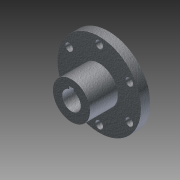
# Autodesk Inventor part: wheel hub
Saved by Autodesk Inventor 2011 SP1 (Build 150282100, 282)
## iProperties
Created: 2012-01-20
Part Number: wheel hub
Document SubType Name: Modeling
Designer: Christopher
Density: 1 g/cm^3
Author: Christopher
Autodesk Inventor part; units mm, degrees
ref_plane "YZ Plane" through (0, 0, 0) normal (1, 0, 0) x (0, 1, 0)
ref_plane "XZ Plane" through (0, 0, 0) normal (0, 1, 0) x (-1, 0, 0)
ref_plane "XY Plane" through (0, 0, 0) normal (0, 0, 1) x (1, 0, 0)
sketch "Sketch1" plane through (0, 0, 0) normal (0, 0, 1) x (1, 0, 0)
  circle A0 centre (0, 0) radius 28.575
  circle A1 centre (0, 0) radius 6.35
  line L0 (-1.5875, 4.7625) -> (1.5875, 4.7625)
  line L1 (1.5875, 4.7625) -> (1.5875, 7.9375)
  line L2 (1.5875, 7.9375) -> (-1.5875, 7.9375)
  line L3 (-1.5875, 7.9375) -> (-1.5875, 4.7625)
  line L4 (1.5875, 6.35) -> (-1.5875, 6.35)
  circle A2 centre (0, 0) radius 12.7
  point P0 (0, 4.7625)
  point P1 (0, 23.8125)
  point P2 (-20.6222, 11.9063)
  point P3 (-20.6222, -11.9062)
  point P4 (0, -23.8125)
  point P5 (20.6222, -11.9063)
  point P6 (20.6222, 11.9062)
  dimension "d0" = 57.15
  dimension "d1" = 12.7
  dimension "d2" = 3.175
  dimension "d3" = 3.175
  dimension "d6" = 360
  dimension "d8" = 23.8125
  dimension "d9" = 25.4
  constraints: 10 end point, 5 coincident, 3 centre point, 3 midpoint, 2 parallel, 1 horizontal, 1 perpendicular, 1 tangent, 1 vertical alignment, 11 other
  measures "d0" diameter of A0
  measures "d1" diameter of A1
  measures "d2" distance of L0.end L1.end
  measures "d3" distance of L1.end L2.end
  measures "d8" distance of point (0, 0) point (0, 23.812)
  measures "d9" diameter of A2
extrude "Extrusion1" add sketch "Sketch1" against normal blind 6.35 contours A0 | A2
extrude "Extrusion2" add sketch "Sketch1" along normal blind 19.05 contours A2
hole "Hole1" at (0, 23.8125, 0) at (-20.6222, 11.9063, 0) at (-20.6222, -11.9062, 0) at (0, -23.8125, 0) at (20.6222, -11.9063, 0) at (20.6222, 11.9062, 0) direction (0, 0, -1) diameter 5.1816 depth 25.4 tip angle 118
body "Solid1"
